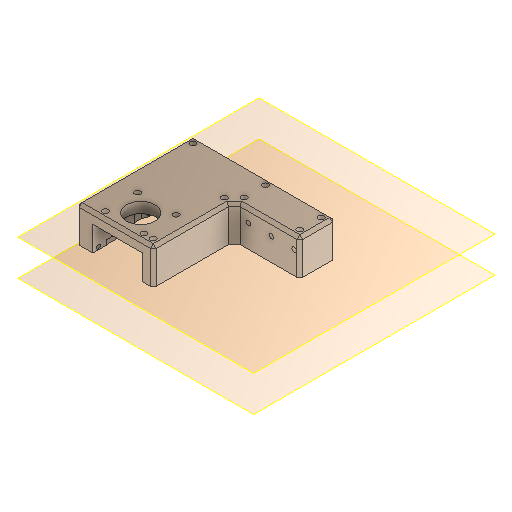
# Autodesk Inventor part: MIAB_Case_v0
Saved by Autodesk Inventor 2024.1 (Build 281209000, 209)
## iProperties
Created: 2024-08-15
Part Number: MIAB_Case_v0
Material: Generisch
Document SubType Name: Modeling
Designer: diederichbenedict
Density: 1 g/cm^3
Appearance: Vorgabe
Author: diederichbenedict
Autodesk Inventor part; units mm, degrees
ref_plane "YZ Plane" through (0, 0, 0) normal (1, 0, 0) x (0, 1, 0)
ref_plane "XZ Plane" through (0, 0, 0) normal (0, 1, 0) x (-1, 0, 0)
ref_plane "XY Plane" through (0, 0, 0) normal (0, 0, 1) x (1, 0, 0)
ref_plane "Arbeitsebene2" through (0, 0, 25) normal (0, 0, 1) x (1, 0, 0)
ref_plane "Arbeitsebene1" through (0, 0, 0) normal (0, 0, 1) x (1, 0, 0)
sketch "Skizze1" plane through (0, 0, 25) normal (0, 0, 1) x (1, 0, 0)
  line L0 (-13.8965, 67) -> (-13.9983, 78.6618) construction
  line L1 (13.8965, 67) -> (13.9983, 78.662) construction
  line L2 (19.5, 77) -> (19.5, 27) construction
  line L3 (-21, 25) -> (21, 25) construction
  line L4 (-13.5, -5.43) -> (-13.5, -26.78) construction
  line L5 (13.5, -5.43) -> (13.5, -26.78) construction
  line L6 (71, 52) -> (31, 52) construction
  line L7 (-29, -4.93) -> (-29, 77)
  line L8 (-29, 77) -> (71, 77)
  line L9 (71, 77) -> (71, 52)
  line L10 (71, 52) -> (29, 52)
  line L11 (29, 52) -> (25, 48)
  line L12 (25, 48) -> (25, -4.93)
  line L13 (25, -4.93) -> (-29, -4.93)
  line L14 (-12.225, -4.93) -> (12.225, -4.93) projected
  line L15 (-19.5, 77) -> (19.5, 77) projected
  point P0 (0, 0)
  dimension "d1" = 135
  dimension "d2" = 8
  dimension "d3" = 0
  dimension "d4" = 4
  dimension "d5" = 4
  dimension "d6" = 0
  constraints: 24 end point, 4 vertical, 2 parallel, 2 perpendicular, 1 point on line, 13 other
  measures "d1" angle of L11 L10
  measures "d2" distance from line of L7 L3.start
  measures "d3" distance between parallel lines of L14 L13
  measures "d4" distance from line of L12 L3.end
  measures "d5" horizontal distance of L11.end L10.end
  measures "d6" vertical extent of L8
extrude "Extrusion1" add sketch "Skizze1" against normal up to surface (25 mm away)
sketch "Skizze2" plane through (71, 77, 0) normal (0, 0, -1) x (-1, 0, 0)
  line L0 (81.08, -67) -> (81.08, -71.93)
  line L1 (92, -44) -> (92, -52)
  line L2 (90.5, -40) -> (92, -44)
  line L3 (90.5, 0) -> (90.5, -40)
  line L4 (50, -52) -> (92, -52) construction
  line L5 (71, 10.4) -> (71, -62.4)
  line L6 (100, -81.93) -> (46, -81.93) projected
  line L7 (53.5, -72.07) -> (88.5, -72.07)
  line L8 (88.5, -72.07) -> (88.5, -81.93)
  line L9 (88.5, -81.93) -> (53.5, -81.93)
  line L10 (53.5, -81.93) -> (53.5, -72.07)
  line L11 (53.5, -72.07) -> (88.5, -81.93) construction
  line L12 (88.5, -72.07) -> (53.5, -81.93) construction
  line L13 (88.5, -72.07) -> (88.5, -52)
  line L14 (71, -81.93) -> (71, 0)
  line L15 (71, 0) -> (90.5, 0)
  line L16 (92, -52) -> (88.5, -52)
  line L17 (88.8, -72.07) -> (88.8, -52.3)
  line L18 (88.8, -52.3) -> (92.3, -52.3)
  line L19 (92.3, -52.3) -> (92.3, -43.9456)
  line L20 (92.3, -43.9456) -> (90.8, -39.9456)
  line L21 (90.8, -39.9456) -> (90.8, 0.3)
  line L22 (90.8, 0.3) -> (70.7, 0.3)
  line L23 (70.7, 0.3) -> (70.7, -81.93)
  line L24 (88.8, -72.07) -> (88.5, -72.07)
  line L25 (90.8, -1.4268) -> (89.8018, 0.3)
  point P0 (71, -77)
  point P1 (46, -81.93)
  point P2 (71, -81.93)
  point P3 (71, 0.3)
  dimension "d9" = 35
  dimension "d34" = 0.3
  constraints: 48 end point, 4 perpendicular, 4 point on line, 4 vertical, 3 midpoint, 2 horizontal, 2 parallel, 1 collinear, 17 other
  measures "d9" distance of L8.end L9.end
  measures "d34" distance between parallel lines of L1 L19
revolve "Umdrehung1" cut sketch "Skizze2" angle 360 about axis through (0, -4.93, 0) along (0, 1, 0) contours L2 L3 L25 L21 L20 L19 L18 L17 L24 L13 L16 L1 | L1 L16 L13 L7 L14 L5 L15 L25 L3 L2 | L8 L6 L14 L7 | L15 L5 L22 L25
chamfer "Fasen1" distance 2 angle 45 12 edges at (-29, -4.93, 12.5) (-29, 36.035, 25) (-29, 77, 12.5) (21, 77, 25) (71, 77, 12.5) (71, 64.5, 25) (71, 52, 12.5) (25, -4.93, 12.5) (-2, -4.93, 25) (25, 21.535, 25) (27, 50, 25) (50, 52, 25)
sketch "Skizze3" plane through (0, 0, 25) normal (0, 0, 1) x (1, 0, 0)
  line L0 (23, -2.93) -> (-27, -2.93) projected
  line L1 (23, 48.8284) -> (23, -2.93) projected
  line L2 (28.1716, 54) -> (23, 48.8284) projected
  line L3 (69, 54) -> (28.1716, 54) projected
  line L4 (69, 75) -> (69, 54) projected
  line L5 (-27, 75) -> (69, 75) projected
  line L6 (-27, -2.93) -> (-27, 75) projected
  line L7 (66, 57) -> (26.9289, 57)
  line L8 (26.9289, 57) -> (20, 50.0711)
  line L9 (20, 50.0711) -> (20, 0.07)
  line L10 (20, 0.07) -> (-24, 0.07)
  line L11 (-24, 0.07) -> (-24, 72)
  line L12 (-24, 72) -> (66, 72)
  line L13 (66, 72) -> (66, 57)
  line L14 (-29, -2.93) -> (-27, -4.93) projected
  line L15 (-29, -2.93) -> (-29, 75) projected
  line L16 (-27, 77) -> (-29, 75) projected
  line L17 (18.9752, 77) -> (69, 77) projected
  line L18 (-17.5, -4.93) -> (-27, -4.93) projected
  line L19 (23, -4.93) -> (25, -2.93) projected
  line L20 (23, -4.93) -> (17.5, -4.93) projected
  line L21 (18.9752, 77) -> (69, 77) projected
  line L22 (71, 75) -> (69, 77) projected
  line L23 (71, 75) -> (71, 54) projected
  line L24 (69, 52) -> (71, 54) projected
  line L25 (69, 52) -> (29, 52) projected
  line L26 (29, 52) -> (25, 48) projected
  line L27 (25, 48) -> (25, -2.93) projected
  line L28 (13.5, 0.07) -> (-13.5, 0.07)
  line L29 (-13.5, 0.07) -> (-13.5, 22.57)
  line L30 (-13.5, 22.57) -> (13.5, 22.57)
  line L31 (13.5, 22.57) -> (13.5, 0.07)
  line L32 (-29, -2.93) -> (-27, -4.93) projected
  line L33 (-29, -2.93) -> (-29, 75) projected
  line L34 (-27, 77) -> (-29, 75) projected
  line L35 (71, 75) -> (69, 77) projected
  line L36 (71, 75) -> (71, 54) projected
  line L37 (69, 52) -> (71, 54) projected
  line L38 (69, 52) -> (29, 52) projected
  line L39 (29, 52) -> (25, 48) projected
  line L40 (25, 48) -> (25, -2.93) projected
  line L41 (23, -4.93) -> (25, -2.93) projected
  line L42 (-27, 77) -> (-18.9752, 77) projected
  line L43 (-19.8, 75.5732) -> (-19.8, 37.0544) projected
  line L44 (-19.8, 37.0544) -> (-21.3, 33.0544) projected
  line L45 (-21.3, 33.0544) -> (-21.3, 24.7) projected
  line L46 (-21.3, 24.7) -> (-17.8, 24.7) projected
  line L47 (-17.8, 24.7) -> (-17.8, 4.93) projected
  line L48 (-17.8, 4.93) -> (-17.5, 4.93) projected
  line L49 (-17.5, 4.93) -> (-17.5, -4.93) projected
  line L50 (-17.5, -4.93) -> (-27, -4.93) projected
  line L51 (17.5, -4.93) -> (17.5, 4.93) projected
  line L52 (17.5, 4.93) -> (17.8, 4.93) projected
  line L53 (17.8, 4.93) -> (17.8, 24.7) projected
  line L54 (17.8, 24.7) -> (21.3, 24.7) projected
  line L55 (21.3, 24.7) -> (21.3, 33.0544) projected
  line L56 (21.3, 33.0544) -> (19.8, 37.0544) projected
  line L57 (19.8, 37.0544) -> (19.8, 75.5732) projected
  line L58 (-27, 77) -> (-18.9752, 77) projected
  line L59 (-19.8, 75.5732) -> (-19.8, 37.0544) projected
  line L60 (-19.8, 37.0544) -> (-21.3, 33.0544) projected
  line L61 (-21.3, 33.0544) -> (-21.3, 24.7) projected
  line L62 (-21.3, 24.7) -> (-17.8, 24.7) projected
  line L63 (-17.8, 24.7) -> (-17.8, 4.93) projected
  line L64 (-17.8, 4.93) -> (-17.5, 4.93) projected
  line L65 (-17.5, 4.93) -> (-17.5, -4.93) projected
  line L66 (23, -4.93) -> (17.5, -4.93) projected
  line L67 (17.5, -4.93) -> (17.5, 4.93) projected
  line L68 (17.5, 4.93) -> (17.8, 4.93) projected
  line L69 (17.8, 4.93) -> (17.8, 24.7) projected
  line L70 (17.8, 24.7) -> (21.3, 24.7) projected
  line L71 (21.3, 24.7) -> (21.3, 33.0544) projected
  line L72 (21.3, 33.0544) -> (19.8, 37.0544) projected
  line L73 (19.8, 37.0544) -> (19.8, 75.5732) projected
  line L74 (-18.9752, 77) -> (-19.8, 75.5732) projected
  line L75 (19.8, 75.5732) -> (18.9752, 77) projected
  line L76 (-18.9752, 77) -> (-19.8, 75.5732) projected
  line L77 (19.8, 75.5732) -> (18.9752, 77) projected
  point P0 (0, 0)
  point P1 (26.9289, 72)
  point P2 (-13.5, 0.07)
  dimension "d14" = 3
  dimension "d26" = 22.5
  constraints: 22 end point, 7 coincident, 3 point on line, 2 parallel, 1 horizontal, 1 perpendicular, 6 other
  measures "d14" distance between parallel lines of L4 L13
  measures "d26" distance of L28.end L29.end
hole "Bohrung1" at (26.9289, 72, 25) at (26.9289, 57, 25) at (66, 57, 25) at (66, 72, 25) at (20, 50.0711, 25) at (20, 0.07, 25) at (-24, 72, 25) at (-13.5, 0.07, 25) at (13.5, 0.07, 25) at (13.5, 22.57, 25) at (-13.5, 22.57, 25) direction (0, 0, -1) diameter 3.2 end through all counterbore diameter 4 counterbore depth 6
sketch "Skizze4" plane through (0, -4.93, 0) normal (0, -1, 0) x (1, 0, 0)
  arc A0 (17.5, 0) -> (-17.5, 0) centre (0, 0) ccw projected
  line L0 (17.5, -17.5) -> (-17.5, -17.5)
  line L1 (-17.5, -17.5) -> (-17.5, 17.5)
  line L2 (-17.5, 17.5) -> (17.5, 17.5)
  line L3 (17.5, 17.5) -> (17.5, -17.5)
  line L4 (17.5, -17.5) -> (-17.5, 17.5) construction
  line L5 (-17.5, -17.5) -> (17.5, 17.5) construction
  point P0 (0, 0)
  constraints: 12 end point, 2 midpoint, 2 parallel, 1 horizontal, 1 perpendicular
extrude "Extrusion2" cut sketch "Skizze4" against normal blind 35
sketch "Skizze5" plane through (0, 77, 0) normal (0, 1, 0) x (1, 0, 0)
  line L0 (31, -20) -> (71, -20) projected
  line L1 (71, -20) -> (71, 20) projected
  line L2 (71, 20) -> (31, 20) projected
  line L3 (31, 20) -> (31, -20) projected
  circle A0 centre (51, 0) radius 1.5 projected
  circle A1 centre (51, -16) radius 1.5 projected
  circle A2 centre (67, -16) radius 1.5 projected
  circle A3 centre (67, 0) radius 1.5 projected
  circle A4 centre (67, 16) radius 1.5 projected
  circle A5 centre (51, 16) radius 1.5 projected
  circle A6 centre (35, 16) radius 1.5 projected
  circle A7 centre (35, 0) radius 1.5 projected
  circle A8 centre (35, -16) radius 1.5 projected
  circle A9 centre (62.5, -11) radius 1.5 projected
  point P0 (0, 0)
hole "Bohrung2" at (35, 77, 16) at (51, 77, 16) at (67, 77, 16) direction (0, -1, 0) diameter 3.2 end through all counterbore diameter 6.5 counterbore depth 16
sketch "Skizze6" plane through (-29, -2.93, 0) normal (-1, 0, 0) x (0, 0, 1)
  line L0 (0, 77.93) -> (23, 77.93) projected
  line L1 (0, 0) -> (0, 77.93) projected
  line L2 (23, 0) -> (0, 0) projected
  line L3 (23, 77.93) -> (23, 0) projected
  line L4 (2, 2) -> (2, 75.93)
  line L5 (2, 75.93) -> (21, 75.93)
  line L6 (21, 75.93) -> (21, 2)
  line L7 (21, 2) -> (2, 2)
  line L8 (-116.1474, 27.13) -> (52.8412, 27.13)
  line L9 (0, 39.9844) -> (19.8, 39.9844) projected
  point P0 (0, 2.93)
  point P1 (21, 39.9844)
  point P2 (2, 39.9844)
  dimension "d35" = 2
  constraints: 10 end point, 4 coincident, 3 point on line, 1 horizontal, 5 other
  measures "d35" distance between parallel lines of L2 L7
hole "Bohrung3" at (-29, -0.93, 21) at (-29, -0.93, 2) at (-29, 73, 21) at (-29, 73, 2) at (-29, 37.0544, 21) at (-29, 37.0544, 2) direction (1, 0, 0) diameter 2.8 depth 20
sketch "Skizze7" plane through (0, 0, 25) normal (0, 0, 1) x (1, 0, 0)
  line L0 (-16, 0) -> (15, 0) projected
  circle A0 centre (-13.5, 22.57) radius 2 projected
  circle A1 centre (13.5, 22.57) radius 2 projected
  circle A2 centre (13.5, 0.07) radius 2 projected
  circle A3 centre (-13.5, 0.07) radius 2 projected
  circle A4 centre (-24, 72) radius 2 projected
  circle A5 centre (20, 0.07) radius 2 projected
  circle A6 centre (20, 50.0711) radius 2 projected
  circle A7 centre (66, 72) radius 2 projected
  circle A8 centre (66, 57) radius 2 projected
  circle A9 centre (26.9289, 57) radius 2 projected
  circle A10 centre (26.9289, 72) radius 2 projected
  line L1 (23, -2.93) -> (-27, -2.93) projected
  line L2 (23, 48.8284) -> (23, -2.93) projected
  line L3 (28.1716, 54) -> (23, 48.8284) projected
  line L4 (69, 54) -> (28.1716, 54) projected
  line L5 (69, 75) -> (69, 54) projected
  line L6 (-27, 75) -> (69, 75) projected
  line L7 (-27, -2.93) -> (-27, 75) projected
  line L8 (13.5, 0.07) -> (-13.5, 0.07)
  line L9 (-13.5, 0.07) -> (-13.5, 22.57)
  line L10 (-13.5, 22.57) -> (13.5, 22.57)
  line L11 (13.5, 22.57) -> (13.5, 0.07)
  circle A11 centre (0, 11.32) radius 10
  point P0 (0, 0)
  dimension "d43" = 20
  constraints: 8 end point, 2 parallel, 1 centre point, 1 horizontal, 1 perpendicular
  measures "d43" diameter of A11
extrude "Extrusion3" cut sketch "Skizze7" against normal blind 35 contours A11
